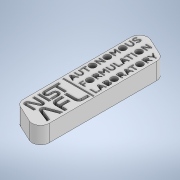
# Autodesk Inventor part: AFL Logo Deskblock
Saved by Autodesk Inventor 2020 (Build 240168000, 168)
## iProperties
Created: 2022-10-06
Part Number: AFL Logo Deskblock
Material: Generic
Document SubType Name: Modeling
Designer: Beaucage
Density: 1 g/cm^3
Appearance: Default
Author: Beaucage
Autodesk Inventor part; units mm, degrees
(part 1 of 4)
ref_plane "YZ Plane" through (0, 0, 0) normal (1, 0, 0) x (0, 1, 0)
ref_plane "XZ Plane" through (0, 0, 0) normal (0, 1, 0) x (-1, 0, 0)
ref_plane "XY Plane" through (0, 0, 0) normal (0, 0, 1) x (1, 0, 0)
sketch "Sketch1" plane through (0, 0, 0) normal (0, 1, 0) x (-1, 0, 0)
  line L0 (3.752764, -91.883884) -> (3.752764, -90.119995)
  line L1 (3.752764, -90.119995) -> (49.613875, -90.119995)
  line L2 (49.613875, -90.119995) -> (49.613875, -91.883884)
  line L3 (49.613875, -91.883884) -> (3.752764, -91.883884)
  line L4 (6.397815, -27.471543) -> (6.397815, -23.344146)
  line L5 (6.395755, -23.334329) -> (25.445066, -30.858762)
  spline S0 degree 3 poles (25.445066, -30.858762) (27.445116, -31.652512) (28.209231, -33.122705) (28.209231, -35.376831) (28.209231, -37.599262) (27.447176, -39.05981) (25.447126, -39.821693) knots 2 2 2 2 3 3 3 4 4 4 4
  line L6 (25.445066, -30.858762) -> (27.445116, -31.652512) construction
  line L7 (27.445116, -31.652512) -> (28.209231, -33.122705) construction
  line L8 (28.209231, -33.122705) -> (28.209231, -35.376831) construction
  line L9 (28.209231, -35.376831) -> (28.209231, -37.599262) construction
  line L10 (28.209231, -37.599262) -> (27.447176, -39.05981) construction
  line L11 (27.447176, -39.05981) -> (25.447126, -39.821693) construction
  line L12 (25.447126, -39.821693) -> (6.397815, -47.060356)
  line L13 (6.397815, -47.060356) -> (6.397815, -42.901264)
  line L14 (6.397815, -42.901264) -> (23.637417, -36.39279)
  spline S1 degree 3 poles (23.637417, -36.39279) (24.145569, -36.202276) (24.367778, -35.853116) (24.367778, -35.345136) (24.367778, -34.837157) (24.145569, -34.487996) (23.637417, -34.265616) knots 7 7 7 7 8 8 8 9 9 9 9
  line L15 (23.637417, -36.39279) -> (24.145569, -36.202276) construction
  line L16 (24.145569, -36.202276) -> (24.367778, -35.853116) construction
  line L17 (24.367778, -35.853116) -> (24.367778, -35.345136) construction
  line L18 (24.367778, -35.345136) -> (24.367778, -34.837157) construction
  line L19 (24.367778, -34.837157) -> (24.145569, -34.487996) construction
  line L20 (24.145569, -34.487996) -> (23.637417, -34.265616) construction
  line L21 (23.637417, -34.265616) -> (6.397815, -27.471543)
  line L22 (27.83068, -66.850936) -> (24.084311, -66.850936)
  line L23 (24.084311, -66.850936) -> (24.084311, -58.215288)
  spline S2 degree 3 poles (24.084311, -58.215288) (24.084311, -54.818251) (22.465116, -53.802293) (20.464893, -53.802293) knots 2 2 2 2 3 3 3 3
  line L24 (24.084311, -58.215288) -> (24.084311, -54.818251) construction
  line L25 (24.084311, -54.818251) -> (22.465116, -53.802293) construction
  line L26 (22.465116, -53.802293) -> (20.464893, -53.802293) construction
  line L27 (20.464893, -53.802293) -> (18.432976, -53.802293)
  line L28 (18.432976, -53.802293) -> (18.432976, -66.723984)
  line L29 (18.432976, -66.723984) -> (14.877293, -66.723984)
  line L30 (14.877293, -66.723984) -> (14.877293, -53.802293)
  line L31 (14.877293, -53.802293) -> (6.400291, -53.802293)
  line L32 (6.400291, -53.802293) -> (6.400291, -50.055923)
  line L33 (6.400291, -50.055923) -> (20.433198, -50.055923)
  spline S3 degree 3 poles (20.433198, -50.055923) (24.719242, -50.055923) (27.83068, -52.278355) (27.83068, -57.961384) knots 10 10 10 10 11 11 11 11
  line L34 (20.433198, -50.055923) -> (24.719242, -50.055923) construction
  line L35 (24.719242, -50.055923) -> (27.83068, -52.278355) construction
  line L36 (27.83068, -52.278355) -> (27.83068, -57.961384) construction
  line L37 (27.83068, -57.961384) -> (27.83068, -66.850936)
  line L38 (27.83068, -74.820476) -> (13.829639, -74.820476)
  spline S4 degree 3 poles (13.829639, -74.820476) (11.766027, -74.820476) (10.146832, -75.836434) (10.146832, -79.201776) knots 1 1 1 1 2 2 2 2
  line L39 (13.829639, -74.820476) -> (11.766027, -74.820476) construction
  line L40 (11.766027, -74.820476) -> (10.146832, -75.836434) construction
  line L41 (10.146832, -75.836434) -> (10.146832, -79.201776) construction
  line L42 (10.146832, -79.201776) -> (10.146832, -87.519959)
  line L43 (10.146832, -87.519959) -> (6.400291, -87.519959)
  line L44 (6.400291, -87.519959) -> (6.400291, -78.979567)
  spline S5 degree 3 poles (6.400291, -78.979567) (6.400291, -73.296538) (9.511901, -71.074107) (13.797945, -71.074107) knots 5 5 5 5 6 6 6 6
  line L45 (6.400291, -78.979567) -> (6.400291, -73.296538) construction
  line L46 (6.400291, -73.296538) -> (9.511901, -71.074107) construction
  line L47 (9.511901, -71.074107) -> (13.797945, -71.074107) construction
  line L48 (13.797945, -71.074107) -> (27.83068, -71.074107)
  line L49 (27.83068, -71.074107) -> (27.83068, -74.820476)
  line L50 (30.386424, -30.462602) -> (30.386424, -27.465197)
  line L51 (30.386424, -27.465197) -> (44.103588, -27.465197)
  spline S6 degree 3 poles (44.103588, -27.465197) (46.338938, -27.465197) (47.837727, -28.735231) (47.837727, -31.402596) (47.837727, -33.790392) (46.618508, -34.857166) (44.662383, -35.568578) knots 2 2 2 2 3 3 3 4 4 4 4
  line L52 (44.103588, -27.465197) -> (46.338938, -27.465197) construction
  line L53 (46.338938, -27.465197) -> (47.837727, -28.735231) construction
  line L54 (47.837727, -28.735231) -> (47.837727, -31.402596) construction
  line L55 (47.837727, -31.402596) -> (47.837727, -33.790392) construction
  line L56 (47.837727, -33.790392) -> (46.618508, -34.857166) construction
  line L57 (46.618508, -34.857166) -> (44.662383, -35.568578) construction
  line L58 (44.662383, -35.568578) -> (33.714042, -40.572752)
  spline S7 degree 3 poles (33.714042, -40.572752) (33.307692, -40.776012) (33.002802, -41.106225) (33.002802, -41.665019) (33.002802, -42.300123) (33.383829, -42.68115) (33.968117, -42.68115) knots 5 5 5 5 6 6 6 7 7 7 7
  line L59 (33.714042, -40.572752) -> (33.307692, -40.776012) construction
  line L60 (33.307692, -40.776012) -> (33.002802, -41.106225) construction
  line L61 (33.002802, -41.106225) -> (33.002802, -41.665019) construction
  line L62 (33.002802, -41.665019) -> (33.002802, -42.300123) construction
  line L63 (33.002802, -42.300123) -> (33.383829, -42.68115) construction
  line L64 (33.383829, -42.68115) -> (33.968117, -42.68115) construction
  line L65 (33.968117, -42.68115) -> (47.532836, -42.68115)
  line L66 (47.532836, -42.68115) -> (47.532836, -45.704049)
  line L67 (47.532836, -45.704049) -> (33.841166, -45.704049)
  spline S8 degree 3 poles (33.841166, -45.704049) (31.580322, -45.704049) (30.081533, -44.408521) (30.081533, -41.766649) (30.081533, -39.378854) (31.300924, -38.286586) (33.256877, -37.575346) knots 10 10 10 10 11 11 11 12 12 12 12
  line L68 (33.841166, -45.704049) -> (31.580322, -45.704049) construction
  line L69 (31.580322, -45.704049) -> (30.081533, -44.408521) construction
  line L70 (30.081533, -44.408521) -> (30.081533, -41.766649) construction
  line L71 (30.081533, -41.766649) -> (30.081533, -39.378854) construction
  line L72 (30.081533, -39.378854) -> (31.300924, -38.286586) construction
  line L73 (31.300924, -38.286586) -> (33.256877, -37.575346) construction
  line L74 (33.256877, -37.575346) -> (44.205219, -32.571001)
  spline S9 degree 3 poles (44.205219, -32.571001) (44.713198, -32.342419) (44.941952, -32.037528) (44.941952, -31.504055) (44.941952, -30.818308) (44.560925, -30.462602) (43.951143, -30.462602) knots 13 13 13 13 14 14 14 15 15 15 15
  line L75 (44.205219, -32.571001) -> (44.713198, -32.342419) construction
  line L76 (44.713198, -32.342419) -> (44.941952, -32.037528) construction
  line L77 (44.941952, -32.037528) -> (44.941952, -31.504055) construction
  line L78 (44.941952, -31.504055) -> (44.941952, -30.818308) construction
  line L79 (44.941952, -30.818308) -> (44.560925, -30.462602) construction
  line L80 (44.560925, -30.462602) -> (43.951143, -30.462602) construction
  line L81 (43.951143, -30.462602) -> (30.386424, -30.462602)
  line L82 (47.757456, -53.402317) -> (30.611044, -53.402317)
  line L83 (30.611044, -53.402317) -> (30.611044, -50.404739)
  line L84 (30.611044, -50.404739) -> (47.757456, -50.404739)
  line L85 (47.757456, -50.404739) -> (47.757456, -53.402317)
  line L86 (47.757456, -69.134173) -> (44.760051, -69.134173)
  line L87 (44.760051, -69.134173) -> (44.760051, -60.344873)
  spline S10 degree 3 poles (44.760051, -60.344873) (44.760051, -58.795442) (43.921859, -58.109523) (42.727962, -58.109523) (41.686337, -58.109523) (40.6957, -58.642996) (40.6957, -60.649764) knots 2 2 2 2 3 3 3 4 4 4 4
  line L88 (44.760051, -60.344873) -> (44.760051, -58.795442) construction
  line L89 (44.760051, -58.795442) -> (43.921859, -58.109523) construction
  line L90 (43.921859, -58.109523) -> (42.727962, -58.109523) construction
  line L91 (42.727962, -58.109523) -> (41.686337, -58.109523) construction
  line L92 (41.686337, -58.109523) -> (40.6957, -58.642996) construction
  line L93 (40.6957, -58.642996) -> (40.6957, -60.649764) construction
  line L94 (40.6957, -60.649764) -> (40.6957, -64.663301)
  spline S11 degree 3 poles (40.6957, -64.663301) (40.6957, -69.337262) (38.104643, -70.429701) (35.640711, -70.429701) (32.744764, -70.429701) (30.611044, -68.880097) (30.611044, -64.968192) knots 5 5 5 5 6 6 6 7 7 7 7
  line L95 (40.6957, -64.663301) -> (40.6957, -69.337262) construction
  line L96 (40.6957, -69.337262) -> (38.104643, -70.429701) construction
  line L97 (38.104643, -70.429701) -> (35.640711, -70.429701) construction
  line L98 (35.640711, -70.429701) -> (32.744764, -70.429701) construction
  line L99 (32.744764, -70.429701) -> (30.611044, -68.880097) construction
  line L100 (30.611044, -68.880097) -> (30.611044, -64.968192) construction
  line L101 (30.611044, -64.968192) -> (30.611044, -55.417009)
  line L102 (30.611044, -55.417009) -> (33.608449, -55.417009)
  line L103 (33.608449, -55.417009) -> (33.608449, -65.069822)
  spline S12 degree 3 poles (33.608449, -65.069822) (33.608449, -66.695562) (34.497628, -67.432124) (35.742341, -67.432124) (36.85993, -67.432124) (37.876061, -66.847836) (37.876061, -64.739609) knots 10 10 10 10 11 11 11 12 12 12 12
  line L104 (33.608449, -65.069822) -> (33.608449, -66.695562) construction
  line L105 (33.608449, -66.695562) -> (34.497628, -67.432124) construction
  line L106 (34.497628, -67.432124) -> (35.742341, -67.432124) construction
  line L107 (35.742341, -67.432124) -> (36.85993, -67.432124) construction
  line L108 (36.85993, -67.432124) -> (37.876061, -66.847836) construction
  line L109 (37.876061, -66.847836) -> (37.876061, -64.739609) construction
  line L110 (37.876061, -64.739609) -> (37.876061, -60.751395)
  spline S13 degree 3 poles (37.876061, -60.751395) (37.876061, -56.179064) (40.441624, -55.112118) (42.82942, -55.112118) (45.674552, -55.112118) (47.757456, -56.636228) (47.757456, -60.446504) knots 13 13 13 13 14 14 14 15 15 15 15
  line L111 (37.876061, -60.751395) -> (37.876061, -56.179064) construction
  line L112 (37.876061, -56.179064) -> (40.441624, -55.112118) construction
  line L113 (40.441624, -55.112118) -> (42.82942, -55.112118) construction
  line L114 (42.82942, -55.112118) -> (45.674552, -55.112118) construction
  line L115 (45.674552, -55.112118) -> (47.757456, -56.636228) construction
  line L116 (47.757456, -56.636228) -> (47.757456, -60.446504) construction
  line L117 (47.757456, -60.446504) -> (47.757456, -69.134173)
  line L118 (47.757456, -82.150088) -> (44.760051, -82.150088)
  line L119 (44.760051, -82.150088) -> (44.760051, -77.145915)
  line L120 (44.760051, -77.145915) -> (30.611044, -77.145915)
  line L121 (30.611044, -77.145915) -> (30.611044, -74.123016)
  line L122 (30.611044, -74.123016) -> (44.760051, -74.123016)
  line L123 (44.760051, -74.123016) -> (44.760051, -69.118843)
  line L124 (44.760051, -69.118843) -> (47.757456, -69.118843)
  line L125 (47.757456, -69.118843) -> (47.757456, -82.150088)
  line L126 (42.092514, -97.973412) -> (40.30072, -97.239779)
  spline S14 degree 3 poles (40.30072, -97.239779) (39.919692, -97.084577) (39.722288, -96.844799) (39.722288, -96.477896) (39.722288, -96.026416) (40.018566, -95.716013) (40.427671, -95.687763) knots 1 1 1 1 2 2 2 3 3 3 3
  line L127 (40.30072, -97.239779) -> (39.919692, -97.084577) construction
  line L128 (39.919692, -97.084577) -> (39.722288, -96.844799) construction
  line L129 (39.722288, -96.844799) -> (39.722288, -96.477896) construction
  line L130 (39.722288, -96.477896) -> (39.722288, -96.026416) construction
  line L131 (39.722288, -96.026416) -> (40.018566, -95.716013) construction
  line L132 (40.018566, -95.716013) -> (40.427671, -95.687763) construction
  spline S15 degree 3 poles (40.427671, -95.687763) (40.611123, -95.673811) (40.780449, -95.730138) (40.977853, -95.814887) knots 3 3 3 3 4 4 4 4
  line L133 (40.427671, -95.687763) -> (40.611123, -95.673811) construction
  line L134 (40.611123, -95.673811) -> (40.780449, -95.730138) construction
  line L135 (40.780449, -95.730138) -> (40.977853, -95.814887) construction
  line L136 (40.977853, -95.814887) -> (48.102827, -98.77767)
  spline S16 degree 3 poles (48.102827, -98.77767) (48.89296, -99.088073) (49.189238, -99.511303) (49.189238, -100.146234) knots 5 5 5 5 6 6 6 6
  line L137 (48.102827, -98.77767) -> (48.89296, -99.088073) construction
  line L138 (48.89296, -99.088073) -> (49.189238, -99.511303) construction
  line L139 (49.189238, -99.511303) -> (49.189238, -100.146234) construction
  line L140 (49.189238, -100.146234) -> (49.189238, -100.244936)
  spline S17 degree 3 poles (49.189238, -100.244936) (49.189238, -100.893992) (48.89296, -101.303097) (48.102827, -101.627625) knots 7 7 7 7 8 8 8 8
  line L141 (49.189238, -100.244936) -> (49.189238, -100.893992) construction
  line L142 (49.189238, -100.893992) -> (48.89296, -101.303097) construction
  line L143 (48.89296, -101.303097) -> (48.102827, -101.627625) construction
  line L144 (48.102827, -101.627625) -> (40.921526, -104.590407)
  spline S18 degree 3 poles (40.921526, -104.590407) (40.738074, -104.661031) (40.582873, -104.703406) (40.470046, -104.703406) (40.032691, -104.703406) (39.722288, -104.350628) (39.722288, -103.885024) (39.722288, -103.546371) (39.933817, -103.264217) (40.314844, -103.109016) knots 9 9 9 9 10 10 10 11 11 11 12 12 12 12
  line L145 (40.921526, -104.590407) -> (40.738074, -104.661031) construction
  line L146 (40.738074, -104.661031) -> (40.582873, -104.703406) construction
  line L147 (40.582873, -104.703406) -> (40.470046, -104.703406) construction
  line L148 (40.470046, -104.703406) -> (40.032691, -104.703406) construction
  line L149 (40.032691, -104.703406) -> (39.722288, -104.350628) construction
  line L150 (39.722288, -104.350628) -> (39.722288, -103.885024) construction
  line L151 (39.722288, -103.885024) -> (39.722288, -103.546371) construction
  line L152 (39.722288, -103.546371) -> (39.933817, -103.264217) construction
  line L153 (39.933817, -103.264217) -> (40.314844, -103.109016) construction
  line L154 (40.314844, -103.109016) -> (42.092514, -102.389508)
  line L155 (42.092514, -102.389508) -> (42.092514, -97.973412)
  line L156 (43.503453, -101.839326) -> (47.637223, -100.216686)
  line L157 (47.637223, -100.216686) -> (47.637223, -100.174484)
  line L158 (47.637223, -100.174484) -> (43.503453, -98.509641)
  line L159 (43.503453, -98.509641) -> (43.503453, -101.839326)
  spline S19 degree 3 poles (41.14718, -110.390914) (41.14718, -111.900555) (42.177091, -112.845889) (43.785606, -112.845889) knots 0 0 0 0 1 1 1 1
  line L160 (41.14718, -110.390914) -> (41.14718, -111.900555) construction
  line L161 (41.14718, -111.900555) -> (42.177091, -112.845889) construction
  line L162 (42.177091, -112.845889) -> (43.785606, -112.845889) construction
  line L163 (43.785606, -112.845889) -> (48.511932, -112.845889)
  spline S20 degree 3 poles (48.511932, -112.845889) (48.92121, -112.845889) (49.203363, -113.170245) (49.203363, -113.621725) (49.203363, -114.073205) (48.92121, -114.397733) (48.511932, -114.397733) knots 2 2 2 2 3 3 3 4 4 4 4
  line L164 (48.511932, -112.845889) -> (48.92121, -112.845889) construction
  line L165 (48.92121, -112.845889) -> (49.203363, -113.170245) construction
  line L166 (49.203363, -113.170245) -> (49.203363, -113.621725) construction
  line L167 (49.203363, -113.621725) -> (49.203363, -114.073205) construction
  line L168 (49.203363, -114.073205) -> (48.92121, -114.397733) construction
  line L169 (48.92121, -114.397733) -> (48.511932, -114.397733) construction
  line L170 (48.511932, -114.397733) -> (43.700857, -114.397733)
  spline S21 degree 3 poles (43.700857, -114.397733) (41.358881, -114.397733) (39.637539, -112.902217) (39.637539, -110.390914) (39.637539, -107.865487) (41.358881, -106.383924) (43.700857, -106.383924) knots 5 5 5 5 6 6 6 7 7 7 7
  line L171 (43.700857, -114.397733) -> (41.358881, -114.397733) construction
  line L172 (41.358881, -114.397733) -> (39.637539, -112.902217) construction
  line L173 (39.637539, -112.902217) -> (39.637539, -110.390914) construction
  line L174 (39.637539, -110.390914) -> (39.637539, -107.865487) construction
  line L175 (39.637539, -107.865487) -> (41.358881, -106.383924) construction
  line L176 (41.358881, -106.383924) -> (43.700857, -106.383924) construction
  line L177 (43.700857, -106.383924) -> (48.511932, -106.383924)
  spline S22 degree 3 poles (48.511932, -106.383924) (48.92121, -106.383924) (49.203363, -106.708452) (49.203363, -107.159931) (49.203363, -107.611411) (48.92121, -107.935939) (48.511932, -107.935939) knots 8 8 8 8 9 9 9 10 10 10 10
  line L178 (48.511932, -106.383924) -> (48.92121, -106.383924) construction
  line L179 (48.92121, -106.383924) -> (49.203363, -106.708452) construction
  line L180 (49.203363, -106.708452) -> (49.203363, -107.159931) construction
  line L181 (49.203363, -107.159931) -> (49.203363, -107.611411) construction
  line L182 (49.203363, -107.611411) -> (48.92121, -107.935939) construction
  line L183 (48.92121, -107.935939) -> (48.511932, -107.935939) construction
  line L184 (48.511932, -107.935939) -> (43.785606, -107.935939)
  spline S23 degree 3 poles (43.785606, -107.935939) (42.191216, -107.935939) (41.14718, -108.867148) (41.14718, -110.390914) knots 11 11 11 11 12 12 12 12
  line L185 (43.785606, -107.935939) -> (42.191216, -107.935939) construction
  line L186 (42.191216, -107.935939) -> (41.14718, -108.867148) construction
  line L187 (41.14718, -108.867148) -> (41.14718, -110.390914) construction
  spline S24 degree 3 poles (48.384981, -115.895143) (48.83646, -115.895143) (49.104489, -116.191421) (49.104489, -116.657026) knots 0 0 0 0 1 1 1 1
  line L188 (48.384981, -115.895143) -> (48.83646, -115.895143) construction
  line L189 (48.83646, -115.895143) -> (49.104489, -116.191421) construction
  line L190 (49.104489, -116.191421) -> (49.104489, -116.657026) construction
  line L191 (49.104489, -116.657026) -> (49.104489, -123.866577)
  spline S25 degree 3 poles (49.104489, -123.866577) (49.104489, -124.33201) (48.83646, -124.614163) (48.384981, -124.614163) (47.947626, -124.614163) (47.679597, -124.33201) (47.679597, -123.866577) knots 2 2 2 2 3 3 3 4 4 4 4
  line L192 (49.104489, -123.866577) -> (49.104489, -124.33201) construction
  line L193 (49.104489, -124.33201) -> (48.83646, -124.614163) construction
  line L194 (48.83646, -124.614163) -> (48.384981, -124.614163) construction
  line L195 (48.384981, -124.614163) -> (47.947626, -124.614163) construction
  line L196 (47.947626, -124.614163) -> (47.679597, -124.33201) construction
  line L197 (47.679597, -124.33201) -> (47.679597, -123.866577) construction
  line L198 (47.679597, -123.866577) -> (47.679597, -121.0447)
  line L199 (47.679597, -121.0447) -> (40.413546, -121.0447)
  spline S26 degree 3 poles (40.413546, -121.0447) (40.004441, -121.0447) (39.722288, -120.720172) (39.722288, -120.268864) (39.722288, -119.817212) (40.004441, -119.492684) (40.413546, -119.492684) knots 6 6 6 6 7 7 7 8 8 8 8
  line L200 (40.413546, -121.0447) -> (40.004441, -121.0447) construction
  line L201 (40.004441, -121.0447) -> (39.722288, -120.720172) construction
  line L202 (39.722288, -120.720172) -> (39.722288, -120.268864) construction
  line L203 (39.722288, -120.268864) -> (39.722288, -119.817212) construction
  line L204 (39.722288, -119.817212) -> (40.004441, -119.492684) construction
  line L205 (40.004441, -119.492684) -> (40.413546, -119.492684) construction
  line L206 (40.413546, -119.492684) -> (47.679597, -119.492684)
  line L207 (47.679597, -119.492684) -> (47.679597, -116.642901)
  spline S27 degree 3 poles (47.679597, -116.642901) (47.679597, -116.191421) (47.947626, -115.895143) (48.384981, -115.895143) knots 10 10 10 10 11 11 11 11
  line L208 (47.679597, -116.642901) -> (47.679597, -116.191421) construction
  line L209 (47.679597, -116.191421) -> (47.947626, -115.895143) construction
  line L210 (47.947626, -115.895143) -> (48.384981, -115.895143) construction
  spline S28 degree 3 poles (44.476864, -125.067193) (47.256367, -125.067193) (49.25969, -127.211765) (49.25969, -130.005049) (49.25969, -132.798677) (47.256367, -134.957373) (44.476864, -134.957373) (41.683409, -134.957373) (39.665788, -132.798677) (39.665788, -130.005049) (39.665788, -127.211765) (41.683409, -125.067193) (44.476864, -125.067193) knots 0 0 0 0 1 1 1 2 2 2 3 3 3 4 4 4 4
  line L211 (44.476864, -125.067193) -> (47.256367, -125.067193) construction
  line L212 (47.256367, -125.067193) -> (49.25969, -127.211765) construction
  line L213 (49.25969, -127.211765) -> (49.25969, -130.005049) construction
  line L214 (49.25969, -130.005049) -> (49.25969, -132.798677) construction
  line L215 (49.25969, -132.798677) -> (47.256367, -134.957373) construction
  line L216 (47.256367, -134.957373) -> (44.476864, -134.957373) construction
  line L217 (44.476864, -134.957373) -> (41.683409, -134.957373) construction
  line L218 (41.683409, -134.957373) -> (39.665788, -132.798677) construction
  line L219 (39.665788, -132.798677) -> (39.665788, -130.005049) construction
  line L220 (39.665788, -130.005049) -> (39.665788, -127.211765) construction
  line L221 (39.665788, -127.211765) -> (41.683409, -125.067193) construction
  line L222 (41.683409, -125.067193) -> (44.476864, -125.067193) construction
  spline S29 degree 3 poles (41.189554, -130.005049) (41.189554, -131.740688) (42.431167, -133.264109) (44.462739, -133.264109) (46.494484, -133.264109) (47.735925, -131.740688) (47.735925, -130.005049) (47.735925, -128.283879) (46.494484, -126.760113) (44.462739, -126.760113) (42.431167, -126.760113) (41.189554, -128.283879) (41.189554, -130.005049) knots 0 0 0 0 1 1 1 2 2 2 3 3 3 4 4 4 4
  line L223 (41.189554, -130.005049) -> (41.189554, -131.740688) construction
  line L224 (41.189554, -131.740688) -> (42.431167, -133.264109) construction
  line L225 (42.431167, -133.264109) -> (44.462739, -133.264109) construction
  line L226 (44.462739, -133.264109) -> (46.494484, -133.264109) construction
  line L227 (46.494484, -133.264109) -> (47.735925, -131.740688) construction
  line L228 (47.735925, -131.740688) -> (47.735925, -130.005049) construction
  line L229 (47.735925, -130.005049) -> (47.735925, -128.283879) construction
  line L230 (47.735925, -128.283879) -> (46.494484, -126.760113) construction
  line L231 (46.494484, -126.760113) -> (44.462739, -126.760113) construction
  line L232 (44.462739, -126.760113) -> (42.431167, -126.760113) construction
  line L233 (42.431167, -126.760113) -> (41.189554, -128.283879) construction
  line L234 (41.189554, -128.283879) -> (41.189554, -130.005049) construction
  line L235 (39.722288, -144.355594) -> (39.722288, -144.299094)
  spline S30 degree 3 poles (39.722288, -144.299094) (39.722288, -143.819192) (39.933817, -143.508789) (40.427671, -143.156356) knots 1 1 1 1 2 2 2 2
  line L236 (39.722288, -144.299094) -> (39.722288, -143.819192) construction
  line L237 (39.722288, -143.819192) -> (39.933817, -143.508789) construction
  line L238 (39.933817, -143.508789) -> (40.427671, -143.156356) construction
  line L239 (40.427671, -143.156356) -> (46.734263, -138.655683)
  line L240 (46.734263, -138.655683) -> (40.413546, -138.655683)
  spline S31 degree 3 poles (40.413546, -138.655683) (40.004441, -138.655683) (39.722288, -138.331155) (39.722288, -137.879503) (39.722288, -137.428196) (40.004441, -137.103668) (40.413546, -137.103668) knots 4 4 4 4 5 5 5 6 6 6 6
  line L241 (40.413546, -138.655683) -> (40.004441, -138.655683) construction
  line L242 (40.004441, -138.655683) -> (39.722288, -138.331155) construction
  line L243 (39.722288, -138.331155) -> (39.722288, -137.879503) construction
  line L244 (39.722288, -137.879503) -> (39.722288, -137.428196) construction
  line L245 (39.722288, -137.428196) -> (40.004441, -137.103668) construction
  line L246 (40.004441, -137.103668) -> (40.413546, -137.103668) construction
  line L247 (40.413546, -137.103668) -> (48.258029, -137.103668)
  spline S32 degree 3 poles (48.258029, -137.103668) (48.822336, -137.103668) (49.189238, -137.484351) (49.189238, -137.964253) knots 7 7 7 7 8 8 8 8
  line L248 (48.258029, -137.103668) -> (48.822336, -137.103668) construction
  line L249 (48.822336, -137.103668) -> (49.189238, -137.484351) construction
  line L250 (49.189238, -137.484351) -> (49.189238, -137.964253) construction
  line L251 (49.189238, -137.964253) -> (49.189238, -138.049002)
  spline S33 degree 3 poles (49.189238, -138.049002) (49.189238, -138.528559) (49.019912, -138.782463) (48.41323, -139.234115) knots 9 9 9 9 10 10 10 10
  line L252 (49.189238, -138.049002) -> (49.189238, -138.528559) construction
  line L253 (49.189238, -138.528559) -> (49.019912, -138.782463) construction
  line L254 (49.019912, -138.782463) -> (48.41323, -139.234115) construction
  line L255 (48.41323, -139.234115) -> (42.29009, -143.734788)
  line L256 (42.29009, -143.734788) -> (48.511932, -143.734788)
  spline S34 degree 3 poles (48.511932, -143.734788) (48.92121, -143.734788) (49.203363, -144.059316) (49.203363, -144.510623) (49.203363, -144.962275) (48.92121, -145.286803) (48.511932, -145.286803) knots 12 12 12 12 13 13 13 14 14 14 14
  line L257 (48.511932, -143.734788) -> (48.92121, -143.734788) construction
  line L258 (48.92121, -143.734788) -> (49.203363, -144.059316) construction
  line L259 (49.203363, -144.059316) -> (49.203363, -144.510623) construction
  line L260 (49.203363, -144.510623) -> (49.203363, -144.962275) construction
  line L261 (49.203363, -144.962275) -> (48.92121, -145.286803) construction
  line L262 (48.92121, -145.286803) -> (48.511932, -145.286803) construction
  line L263 (48.511932, -145.286803) -> (40.554623, -145.286803)
  spline S35 degree 3 poles (40.554623, -145.286803) (40.060769, -145.286803) (39.722288, -144.849276) (39.722288, -144.355594) knots 15 15 15 15 16 16 16 16
  line L264 (40.554623, -145.286803) -> (40.060769, -145.286803) construction
  line L265 (40.060769, -145.286803) -> (39.722288, -144.849276) construction
  line L266 (39.722288, -144.849276) -> (39.722288, -144.355594) construction
  spline S36 degree 3 poles (44.476864, -147.432753) (47.256367, -147.432753) (49.25969, -149.577325) (49.25969, -152.370953) (49.25969, -155.164236) (47.256367, -157.322933) (44.476864, -157.322933) (41.683409, -157.322933) (39.665788, -155.164236) (39.665788, -152.370953) (39.665788, -149.577325) (41.683409, -147.432753) (44.476864, -147.432753) knots 0 0 0 0 1 1 1 2 2 2 3 3 3 4 4 4 4
  line L267 (44.476864, -147.432753) -> (47.256367, -147.432753) construction
  line L268 (47.256367, -147.432753) -> (49.25969, -149.577325) construction
  line L269 (49.25969, -149.577325) -> (49.25969, -152.370953) construction
  line L270 (49.25969, -152.370953) -> (49.25969, -155.164236) construction
  line L271 (49.25969, -155.164236) -> (47.256367, -157.322933) construction
  line L272 (47.256367, -157.322933) -> (44.476864, -157.322933) construction
  line L273 (44.476864, -157.322933) -> (41.683409, -157.322933) construction
  line L274 (41.683409, -157.322933) -> (39.665788, -155.164236) construction
  line L275 (39.665788, -155.164236) -> (39.665788, -152.370953) construction
  line L276 (39.665788, -152.370953) -> (39.665788, -149.577325) construction
  line L277 (39.665788, -149.577325) -> (41.683409, -147.432753) construction
  line L278 (41.683409, -147.432753) -> (44.476864, -147.432753) construction
  spline S37 degree 3 poles (41.189554, -152.370953) (41.189554, -154.106248) (42.431167, -155.630013) (44.462739, -155.630013) (46.494484, -155.630013) (47.735925, -154.106248) (47.735925, -152.370953) (47.735925, -150.649439) (46.494484, -149.126018) (44.462739, -149.126018) (42.431167, -149.126018) (41.189554, -150.649439) (41.189554, -152.370953) knots 0 0 0 0 1 1 1 2 2 2 3 3 3 4 4 4 4
  line L279 (41.189554, -152.370953) -> (41.189554, -154.106248) construction
  line L280 (41.189554, -154.106248) -> (42.431167, -155.630013) construction
  line L281 (42.431167, -155.630013) -> (44.462739, -155.630013) construction
  line L282 (44.462739, -155.630013) -> (46.494484, -155.630013) construction
  line L283 (46.494484, -155.630013) -> (47.735925, -154.106248) construction
  line L284 (47.735925, -154.106248) -> (47.735925, -152.370953) construction
  line L285 (47.735925, -152.370953) -> (47.735925, -150.649439) construction
  line L286 (47.735925, -150.649439) -> (46.494484, -149.126018) construction
  line L287 (46.494484, -149.126018) -> (44.462739, -149.126018) construction
  line L288 (44.462739, -149.126018) -> (42.431167, -149.126018) construction
  line L289 (42.431167, -149.126018) -> (41.189554, -150.649439) construction
  line L290 (41.189554, -150.649439) -> (41.189554, -152.370953) construction
  line L291 (46.706013, -166.890652) -> (43.729106, -164.858735)
  spline S38 degree 3 poles (43.729106, -164.858735) (43.305876, -164.576582) (43.13655, -164.350928) (43.13655, -163.9699) (43.13655, -163.602998) (43.305876, -163.391469) (43.729106, -163.095191) knots 1 1 1 1 2 2 2 3 3 3 3
  line L292 (43.729106, -164.858735) -> (43.305876, -164.576582) construction
  line L293 (43.305876, -164.576582) -> (43.13655, -164.350928) construction
  line L294 (43.13655, -164.350928) -> (43.13655, -163.9699) construction
  line L295 (43.13655, -163.9699) -> (43.13655, -163.602998) construction
  line L296 (43.13655, -163.602998) -> (43.305876, -163.391469) construction
  line L297 (43.305876, -163.391469) -> (43.729106, -163.095191) construction
  line L298 (43.729106, -163.095191) -> (46.706013, -161.063618)
  line L299 (46.706013, -161.063618) -> (46.706013, -161.021243)
  line L300 (46.706013, -161.021243) -> (40.413546, -161.021243)
  spline S39 degree 3 poles (40.413546, -161.021243) (39.990316, -161.021243) (39.722288, -160.696715) (39.722288, -160.245408) (39.722288, -159.793756) (39.990316, -159.469228) (40.413546, -159.469228) knots 6 6 6 6 7 7 7 8 8 8 8
  line L301 (40.413546, -161.021243) -> (39.990316, -161.021243) construction
  line L302 (39.990316, -161.021243) -> (39.722288, -160.696715) construction
  line L303 (39.722288, -160.696715) -> (39.722288, -160.245408) construction
  line L304 (39.722288, -160.245408) -> (39.722288, -159.793756) construction
  line L305 (39.722288, -159.793756) -> (39.990316, -159.469228) construction
  line L306 (39.990316, -159.469228) -> (40.413546, -159.469228) construction
  line L307 (40.413546, -159.469228) -> (48.286279, -159.469228)
  spline S40 degree 3 poles (48.286279, -159.469228) (48.83646, -159.469228) (49.189238, -159.86438) (49.189238, -160.386312) knots 9 9 9 9 10 10 10 10
  line L308 (48.286279, -159.469228) -> (48.83646, -159.469228) construction
  line L309 (48.83646, -159.469228) -> (49.189238, -159.86438) construction
  line L310 (49.189238, -159.86438) -> (49.189238, -160.386312) construction
  line L311 (49.189238, -160.386312) -> (49.189238, -160.499311)
  spline S41 degree 3 poles (49.189238, -160.499311) (49.189238, -161.035368) (48.86471, -161.374021) (48.44148, -161.656174) knots 11 11 11 11 12 12 12 12
  line L312 (49.189238, -160.499311) -> (49.189238, -161.035368) construction
  line L313 (49.189238, -161.035368) -> (48.86471, -161.374021) construction
  line L314 (48.86471, -161.374021) -> (48.44148, -161.656174) construction
  line L315 (48.44148, -161.656174) -> (44.998969, -164.012275)
  line L316 (44.998969, -164.012275) -> (44.998969, -164.0264)
  line L317 (44.998969, -164.0264) -> (48.455605, -166.36872)
  spline S42 degree 3 poles (48.455605, -166.36872) (48.86471, -166.650874) (49.189238, -166.918902) (49.189238, -167.454959) knots 15 15 15 15 16 16 16 16
  line L318 (48.455605, -166.36872) -> (48.86471, -166.650874) construction
  line L319 (48.86471, -166.650874) -> (49.189238, -166.918902) construction
  line L320 (49.189238, -166.918902) -> (49.189238, -167.454959) construction
  line L321 (49.189238, -167.454959) -> (49.189238, -167.567958)
  spline S43 degree 3 poles (49.189238, -167.567958) (49.189238, -168.075765) (48.83646, -168.470918) (48.286279, -168.470918) knots 17 17 17 17 18 18 18 18
  line L322 (49.189238, -167.567958) -> (49.189238, -168.075765) construction
  line L323 (49.189238, -168.075765) -> (48.83646, -168.470918) construction
  line L324 (48.83646, -168.470918) -> (48.286279, -168.470918) construction
  line L325 (48.286279, -168.470918) -> (40.413546, -168.470918)
  spline S44 degree 3 poles (40.413546, -168.470918) (39.990316, -168.470918) (39.722288, -168.14639) (39.722288, -167.694738) (39.722288, -167.24343) (39.990316, -166.918902) (40.413546, -166.918902) knots 19 19 19 19 20 20 20 21 21 21 21
  line L326 (40.413546, -168.470918) -> (39.990316, -168.470918) construction
  line L327 (39.990316, -168.470918) -> (39.722288, -168.14639) construction
  line L328 (39.722288, -168.14639) -> (39.722288, -167.694738) construction
  line L329 (39.722288, -167.694738) -> (39.722288, -167.24343) construction
  line L330 (39.722288, -167.24343) -> (39.990316, -166.918902) construction
  line L331 (39.990316, -166.918902) -> (40.413546, -166.918902) construction
  line L332 (40.413546, -166.918902) -> (46.706013, -166.918902)
  line L333 (46.706013, -166.918902) -> (46.706013, -166.890652)
  spline S45 degree 3 poles (44.476864, -170.617212) (47.256367, -170.617212) (49.25969, -172.761784) (49.25969, -175.555412) (49.25969, -178.34904) (47.256367, -180.507737) (44.476864, -180.507737) (41.683409, -180.507737) (39.665788, -178.34904) (39.665788, -175.555412) (39.665788, -172.761784) (41.683409, -170.617212) (44.476864, -170.617212) knots 0 0 0 0 1 1 1 2 2 2 3 3 3 4 4 4 4
  line L334 (44.476864, -170.617212) -> (47.256367, -170.617212) construction
  line L335 (47.256367, -170.617212) -> (49.25969, -172.761784) construction
  line L336 (49.25969, -172.761784) -> (49.25969, -175.555412) construction
  line L337 (49.25969, -175.555412) -> (49.25969, -178.34904) construction
  line L338 (49.25969, -178.34904) -> (47.256367, -180.507737) construction
  line L339 (47.256367, -180.507737) -> (44.476864, -180.507737) construction
  line L340 (44.476864, -180.507737) -> (41.683409, -180.507737) construction
  line L341 (41.683409, -180.507737) -> (39.665788, -178.34904) construction
  line L342 (39.665788, -178.34904) -> (39.665788, -175.555412) construction
  line L343 (39.665788, -175.555412) -> (39.665788, -172.761784) construction
  line L344 (39.665788, -172.761784) -> (41.683409, -170.617212) construction
  line L345 (41.683409, -170.617212) -> (44.476864, -170.617212) construction
  spline S46 degree 3 poles (41.189554, -175.555412) (41.189554, -177.290707) (42.431167, -178.814472) (44.462739, -178.814472) (46.494484, -178.814472) (47.735925, -177.290707) (47.735925, -175.555412) (47.735925, -173.834242) (46.494484, -172.310477) (44.462739, -172.310477) (42.431167, -172.310477) (41.189554, -173.834242) (41.189554, -175.555412) knots 0 0 0 0 1 1 1 2 2 2 3 3 3 4 4 4 4
  line L346 (41.189554, -175.555412) -> (41.189554, -177.290707) construction
  line L347 (41.189554, -177.290707) -> (42.431167, -178.814472) construction
  line L348 (42.431167, -178.814472) -> (44.462739, -178.814472) construction
  line L349 (44.462739, -178.814472) -> (46.494484, -178.814472) construction
  line L350 (46.494484, -178.814472) -> (47.735925, -177.290707) construction
  line L351 (47.735925, -177.290707) -> (47.735925, -175.555412) construction
  line L352 (47.735925, -175.555412) -> (47.735925, -173.834242) construction
  line L353 (47.735925, -173.834242) -> (46.494484, -172.310477) construction
  line L354 (46.494484, -172.310477) -> (44.462739, -172.310477) construction
  line L355 (44.462739, -172.310477) -> (42.431167, -172.310477) construction
  line L356 (42.431167, -172.310477) -> (41.189554, -173.834242) construction
  line L357 (41.189554, -173.834242) -> (41.189554, -175.555412) construction
  spline S47 degree 3 poles (41.14718, -186.575928) (41.14718, -188.085569) (42.177091, -189.030903) (43.785606, -189.030903) knots 0 0 0 0 1 1 1 1
  line L358 (41.14718, -186.575928) -> (41.14718, -188.085569) construction
  line L359 (41.14718, -188.085569) -> (42.177091, -189.030903) construction
  line L360 (42.177091, -189.030903) -> (43.785606, -189.030903) construction
  line L361 (43.785606, -189.030903) -> (48.511932, -189.030903)
  spline S48 degree 3 poles (48.511932, -189.030903) (48.92121, -189.030903) (49.203363, -189.355431) (49.203363, -189.807083) (49.203363, -190.258391) (48.92121, -190.582919) (48.511932, -190.582919) knots 2 2 2 2 3 3 3 4 4 4 4
  line L362 (48.511932, -189.030903) -> (48.92121, -189.030903) construction
  line L363 (48.92121, -189.030903) -> (49.203363, -189.355431) construction
  line L364 (49.203363, -189.355431) -> (49.203363, -189.807083) construction
  line L365 (49.203363, -189.807083) -> (49.203363, -190.258391) construction
  line L366 (49.203363, -190.258391) -> (48.92121, -190.582919) construction
  line L367 (48.92121, -190.582919) -> (48.511932, -190.582919) construction
  line L368 (48.511932, -190.582919) -> (43.700857, -190.582919)
  spline S49 degree 3 poles (43.700857, -190.582919) (41.358881, -190.582919) (39.637539, -189.087403) (39.637539, -186.575928) (39.637539, -184.050673) (41.358881, -182.569282) (43.700857, -182.569282) knots 5 5 5 5 6 6 6 7 7 7 7
  line L369 (43.700857, -190.582919) -> (41.358881, -190.582919) construction
  line L370 (41.358881, -190.582919) -> (39.637539, -189.087403) construction
  line L371 (39.637539, -189.087403) -> (39.637539, -186.575928) construction
  line L372 (39.637539, -186.575928) -> (39.637539, -184.050673) construction
  line L373 (39.637539, -184.050673) -> (41.358881, -182.569282) construction
  line L374 (41.358881, -182.569282) -> (43.700857, -182.569282) construction
  line L375 (43.700857, -182.569282) -> (48.511932, -182.569282)
  spline S50 degree 3 poles (48.511932, -182.569282) (48.92121, -182.569282) (49.203363, -182.89381) (49.203363, -183.345117) (49.203363, -183.79677) (48.92121, -184.121298) (48.511932, -184.121298) knots 8 8 8 8 9 9 9 10 10 10 10
  line L376 (48.511932, -182.569282) -> (48.92121, -182.569282) construction
  line L377 (48.92121, -182.569282) -> (49.203363, -182.89381) construction
  line L378 (49.203363, -182.89381) -> (49.203363, -183.345117) construction
  line L379 (49.203363, -183.345117) -> (49.203363, -183.79677) construction
  line L380 (49.203363, -183.79677) -> (48.92121, -184.121298) construction
  line L381 (48.92121, -184.121298) -> (48.511932, -184.121298) construction
  line L382 (48.511932, -184.121298) -> (43.785606, -184.121298)
  spline S51 degree 3 poles (43.785606, -184.121298) (42.191216, -184.121298) (41.14718, -185.052162) (41.14718, -186.575928) knots 11 11 11 11 12 12 12 12
  line L383 (43.785606, -184.121298) -> (42.191216, -184.121298) construction
  line L384 (42.191216, -184.121298) -> (41.14718, -185.052162) construction
  line L385 (41.14718, -185.052162) -> (41.14718, -186.575928) construction
  spline S52 degree 3 poles (48.511932, -199.684861) (48.356731, -199.938764) (48.159327, -200.192668) (47.834799, -200.192668) (47.453771, -200.192668) (47.072916, -199.952889) (47.072916, -199.515707) (47.072916, -199.289708) (47.129243, -199.148804) (47.242242, -198.937275) (47.524396, -198.344374) (47.792424, -197.540289) (47.792424, -196.679704) (47.792424, -195.325437) (47.171618, -194.577507) (46.466235, -194.577507) (45.520901, -194.577507) (45.281122, -195.494591) (44.956594, -197.159261) (44.617941, -198.866651) (44.251211, -200.418666) (42.360542, -200.418666) (40.879151, -200.418666) (39.651664, -199.02168) (39.651664, -196.707954) (39.651664, -195.212438) (40.117268, -193.815796) (40.596998, -193.081991) (40.794574, -192.799838) (41.048478, -192.729213) (41.231929, -192.729213) (41.641034, -192.729213) (42.036014, -193.039616) (42.036014, -193.448894) (42.036014, -193.646298) (41.951437, -193.843701) (41.852563, -194.04145) (41.457583, -194.83141) (41.161304, -195.790869) (41.161304, -196.792703) (41.161304, -198.076346) (41.626909, -198.767776) (42.332292, -198.767776) (43.1083, -198.767776) (43.305876, -198.020191) (43.644529, -196.312801) (43.98301, -194.591632) (44.364037, -192.926617) (46.437985, -192.926617) (47.877001, -192.926617) (49.25969, -194.238854) (49.25969, -196.750329) (49.25969, -198.006066) (48.808211, -199.191179) (48.511932, -199.684861) knots 0 0 0 0 1 1 1 2 2 2 3 3 3 4 4 4 5 5 5 6 6 6 7 7 7 8 8 8 9 9 9 10 10 10 11 11 11 12 12 12 13 13 13 14 14 14 15 15 15 16 16 16 17 17 17 18 18 18 18
  line L386 (48.511932, -199.684861) -> (48.356731, -199.938764) construction
  line L387 (48.356731, -199.938764) -> (48.159327, -200.192668) construction
  line L388 (48.159327, -200.192668) -> (47.834799, -200.192668) construction
  line L389 (47.834799, -200.192668) -> (47.453771, -200.192668) construction
  line L390 (47.453771, -200.192668) -> (47.072916, -199.952889) construction
  line L391 (47.072916, -199.952889) -> (47.072916, -199.515707) construction
  line L392 (47.072916, -199.515707) -> (47.072916, -199.289708) construction
  line L393 (47.072916, -199.289708) -> (47.129243, -199.148804) construction
  line L394 (47.129243, -199.148804) -> (47.242242, -198.937275) construction
  line L395 (47.242242, -198.937275) -> (47.524396, -198.344374) construction
  line L396 (47.524396, -198.344374) -> (47.792424, -197.540289) construction
  line L397 (47.792424, -197.540289) -> (47.792424, -196.679704) construction
  line L398 (47.792424, -196.679704) -> (47.792424, -195.325437) construction
  line L399 (47.792424, -195.325437) -> (47.171618, -194.577507) construction
  line L400 (47.171618, -194.577507) -> (46.466235, -194.577507) construction
  line L401 (46.466235, -194.577507) -> (45.520901, -194.577507) construction
  line L402 (45.520901, -194.577507) -> (45.281122, -195.494591) construction
  line L403 (45.281122, -195.494591) -> (44.956594, -197.159261) construction
  line L404 (44.956594, -197.159261) -> (44.617941, -198.866651) construction
  line L405 (44.617941, -198.866651) -> (44.251211, -200.418666) construction
  line L406 (44.251211, -200.418666) -> (42.360542, -200.418666) construction
  line L407 (42.360542, -200.418666) -> (40.879151, -200.418666) construction
  line L408 (40.879151, -200.418666) -> (39.651664, -199.02168) construction
  line L409 (39.651664, -199.02168) -> (39.651664, -196.707954) construction
  line L410 (39.651664, -196.707954) -> (39.651664, -195.212438) construction
  line L411 (39.651664, -195.212438) -> (40.117268, -193.815796) construction
  line L412 (40.117268, -193.815796) -> (40.596998, -193.081991) construction
  line L413 (40.596998, -193.081991) -> (40.794574, -192.799838) construction
  line L414 (40.794574, -192.799838) -> (41.048478, -192.729213) construction
  line L415 (41.048478, -192.729213) -> (41.231929, -192.729213) construction
  line L416 (41.231929, -192.729213) -> (41.641034, -192.729213) construction
  line L417 (41.641034, -192.729213) -> (42.036014, -193.039616) construction
  line L418 (42.036014, -193.039616) -> (42.036014, -193.448894) construction
  line L419 (42.036014, -193.448894) -> (42.036014, -193.646298) construction
  line L420 (42.036014, -193.646298) -> (41.951437, -193.843701) construction
  line L421 (41.951437, -193.843701) -> (41.852563, -194.04145) construction
  line L422 (41.852563, -194.04145) -> (41.457583, -194.83141) construction
  line L423 (41.457583, -194.83141) -> (41.161304, -195.790869) construction
  line L424 (41.161304, -195.790869) -> (41.161304, -196.792703) construction
  line L425 (41.161304, -196.792703) -> (41.161304, -198.076346) construction
  line L426 (41.161304, -198.076346) -> (41.626909, -198.767776) construction
  line L427 (41.626909, -198.767776) -> (42.332292, -198.767776) construction
  line L428 (42.332292, -198.767776) -> (43.1083, -198.767776) construction
  line L429 (43.1083, -198.767776) -> (43.305876, -198.020191) construction
  line L430 (43.305876, -198.020191) -> (43.644529, -196.312801) construction
  line L431 (43.644529, -196.312801) -> (43.98301, -194.591632) construction
  line L432 (43.98301, -194.591632) -> (44.364037, -192.926617) construction
  line L433 (44.364037, -192.926617) -> (46.437985, -192.926617) construction
  line L434 (46.437985, -192.926617) -> (47.877001, -192.926617) construction
  line L435 (47.877001, -192.926617) -> (49.25969, -194.238854) construction
  line L436 (49.25969, -194.238854) -> (49.25969, -196.750329) construction
  line L437 (49.25969, -196.750329) -> (49.25969, -198.006066) construction
  line L438 (49.25969, -198.006066) -> (48.808211, -199.191179) construction
  line L439 (48.808211, -199.191179) -> (48.511932, -199.684861) construction
  line L440 (30.421736, -98.072286) -> (27.938511, -98.072286)
  line L441 (27.938511, -98.072286) -> (27.938511, -101.430049)
  spline S53 degree 3 poles (27.938511, -101.430049) (27.938511, -101.895653) (27.656358, -102.177807) (27.219003, -102.177807) (26.781648, -102.177807) (26.499495, -101.895653) (26.499495, -101.430049) knots 2 2 2 2 3 3 3 4 4 4 4
  line L442 (27.938511, -101.430049) -> (27.938511, -101.895653) construction
  line L443 (27.938511, -101.895653) -> (27.656358, -102.177807) construction
  line L444 (27.656358, -102.177807) -> (27.219003, -102.177807) construction
  line L445 (27.219003, -102.177807) -> (26.781648, -102.177807) construction
  line L446 (26.781648, -102.177807) -> (26.499495, -101.895653) construction
  line L447 (26.499495, -101.895653) -> (26.499495, -101.430049) construction
  line L448 (26.499495, -101.430049) -> (26.499495, -98.072286)
  line L449 (26.499495, -98.072286) -> (23.480041, -98.072286)
  spline S54 degree 3 poles (23.480041, -98.072286) (23.056983, -98.072286) (22.788955, -97.747758) (22.788955, -97.296279) (22.788955, -96.844799) (23.056983, -96.520271) (23.480041, -96.520271) knots 6 6 6 6 7 7 7 8 8 8 8
  line L450 (23.480041, -98.072286) -> (23.056983, -98.072286) construction
  line L451 (23.056983, -98.072286) -> (22.788955, -97.747758) construction
  line L452 (22.788955, -97.747758) -> (22.788955, -97.296279) construction
  line L453 (22.788955, -97.296279) -> (22.788955, -96.844799) construction
  line L454 (22.788955, -96.844799) -> (23.056983, -96.520271) construction
  line L455 (23.056983, -96.520271) -> (23.480041, -96.520271) construction
  line L456 (23.480041, -96.520271) -> (31.508147, -96.520271)
  spline S55 degree 3 poles (31.508147, -96.520271) (31.917252, -96.520271) (32.171155, -96.774174) (32.171155, -97.225654) knots 9 9 9 9 10 10 10 10
  line L457 (31.508147, -96.520271) -> (31.917252, -96.520271) construction
  line L458 (31.917252, -96.520271) -> (32.171155, -96.774174) construction
  line L459 (32.171155, -96.774174) -> (32.171155, -97.225654) construction
  line L460 (32.171155, -97.225654) -> (32.171155, -102.601037)
  spline S56 degree 3 poles (32.171155, -102.601037) (32.171155, -103.066641) (31.903127, -103.348967) (31.451647, -103.348967) (31.014292, -103.348967) (30.746264, -103.066641) (30.746264, -102.615161) knots 11 11 11 11 12 12 12 13 13 13 13
  line L461 (32.171155, -102.601037) -> (32.171155, -103.066641) construction
  line L462 (32.171155, -103.066641) -> (31.903127, -103.348967) construction
  line L463 (31.903127, -103.348967) -> (31.451647, -103.348967) construction
  line L464 (31.451647, -103.348967) -> (31.014292, -103.348967) construction
  line L465 (31.014292, -103.348967) -> (30.746264, -103.066641) construction
  line L466 (30.746264, -103.066641) -> (30.746264, -102.615161) construction
  line L467 (30.746264, -102.615161) -> (30.746264, -98.35444)
  spline S57 degree 3 poles (30.746264, -98.35444) (30.746264, -98.156863) (30.661515, -98.072286) (30.421736, -98.072286) knots 14 14 14 14 15 15 15 15
  line L468 (30.746264, -98.35444) -> (30.746264, -98.156863) construction
  line L469 (30.746264, -98.156863) -> (30.661515, -98.072286) construction
  line L470 (30.661515, -98.072286) -> (30.421736, -98.072286) construction
  spline S58 degree 3 poles (27.543531, -104.027478) (30.323034, -104.027478) (32.326357, -106.17205) (32.326357, -108.965506) (32.326357, -111.758962) (30.323034, -113.917658) (27.543531, -113.917658) (24.750075, -113.917658) (22.732455, -111.758962) (22.732455, -108.965506) (22.732455, -106.17205) (24.750075, -104.027478) (27.543531, -104.027478) knots 0 0 0 0 1 1 1 2 2 2 3 3 3 4 4 4 4
  line L471 (27.543531, -104.027478) -> (30.323034, -104.027478) construction
  line L472 (30.323034, -104.027478) -> (32.326357, -106.17205) construction
  line L473 (32.326357, -106.17205) -> (32.326357, -108.965506) construction
  line L474 (32.326357, -108.965506) -> (32.326357, -111.758962) construction